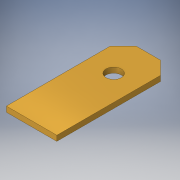
# Autodesk Inventor part: NO_Contact
Saved by Autodesk Inventor 2016 (Build 200138000, 138)
## iProperties
Created: 2016-05-07
Part Number: NO_Contact
Material: Brass, Soft Yellow
Document SubType Name: Modeling
Designer: agmle
Density: 8.47 g/cm^3
Appearance: Brass - Satin
Mass: 0.207764 g
Surface Area: 1.15398 cm^2
Volume: 0.0245294 cm^3
Author: agmle
Autodesk Inventor part; units mm, degrees
ref_plane "YZ Plane" through (0, 0, 0) normal (1, 0, 0) x (0, 1, 0)
ref_plane "XZ Plane" through (0, 0, 0) normal (0, 1, 0) x (-1, 0, 0)
ref_plane "XY Plane" through (0, 0, 0) normal (0, 0, 1) x (1, 0, 0)
sketch "Sketch1" plane through (0, 0, 0) normal (0, 1, 0) x (-1, 0, 0)
  line L0 (0, 0) -> (4.75, 0)
  line L1 (4.75, 0) -> (4.75, -9.75)
  line L2 (3.5, -11) -> (1.25, -11)
  line L3 (0, -9.75) -> (0, 0)
  line L4 (4.75, -9.75) -> (3.5, -11)
  line L5 (1.25, -11) -> (0, -9.75)
  circle A0 centre (2.375, -7.73) radius 0.72
  point P0 (4.75, -11)
  point P1 (0, -11)
  dimension "d0" = 11
  dimension "d1" = 4.75
  dimension "d2" = 1.25
  dimension "d3" = 1.25
  dimension "d4" = 1.25
  dimension "d5" = 1.25
  dimension "d6" = 1.44
  dimension "d7" = 3.27
  constraints: 12 end point, 4 point on line, 2 parallel, 1 centre point, 1 horizontal, 1 perpendicular
  measures "d0" distance between parallel lines of L0 L2
  measures "d1" distance between parallel lines of L3 L1
  measures "d2" distance of L1.end point (4.75, -11)
  measures "d3" distance of L2.start point (4.75, -11)
  measures "d4" distance of L2.end point (0, -11)
  measures "d5" distance of L3.start point (0, -11)
  measures "d6" diameter of A0
  measures "d7" distance from line of L2 A0.centre
extrude "Extrusion1" add sketch "Sketch1" along normal blind 0.5
equation "\"d3\" = d2"
equation "\"d4\" = d2"
equation "\"d5\" = d4"
body "Solid1"
